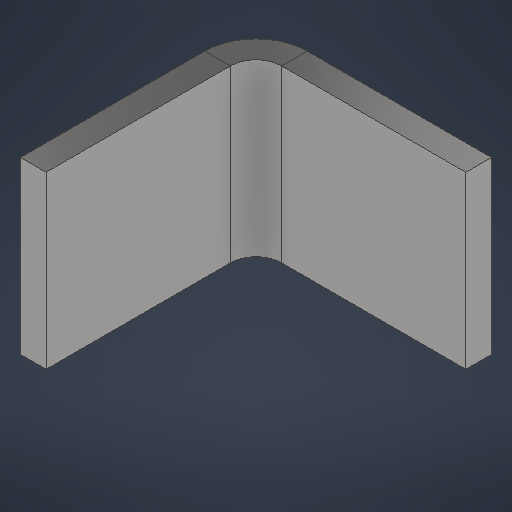
# Autodesk Inventor part: Pressure plate tabs
Saved by Autodesk Inventor 2026.3 (Build 303398000, 398)
## iProperties
Created: 2026-08-04
Part Number: Pressure plate tabs
Material: Generic
Document SubType Name: Sheet Metal
Designer: matot
Density: 1 g/cm^3
Sheet Metal Rule: Default_mm
Appearance: Default
Author: matot
Autodesk Inventor part; units mm, degrees
ref_plane "YZ Plane" through (0, 0, 0) normal (1, 0, 0) x (0, 1, 0)
ref_plane "XZ Plane" through (0, 0, 0) normal (0, 1, 0) x (-1, 0, 0)
ref_plane "XY Plane" through (0, 0, 0) normal (0, 0, 1) x (1, 0, 0)
sketch "Sketch1" plane through (0, 0, 0) normal (1, 0, 0) x (0, 1, 0)
  line L0 (12.963, 18.5185) -> (-7.037, 18.5185)
  line L1 (-7.037, 18.5185) -> (-7.037, -31.4815)
  line L2 (-7.037, -31.4815) -> (12.963, -31.4815)
  line L3 (12.963, -31.4815) -> (12.963, 18.5185)
  point P0 (0, 0)
  dimension "d0" = 50
  dimension "d1" = 20
  measures "d0" distance of L2.end L0.start
  measures "d1" distance of L1.end L2.end
extrude "Plate1" add sketch "Sketch1" along normal blind 3
sketch "Sketch2" plane through (3, 0, 0) normal (1, 0, 0) x (0, 0, -1)
  line L0 (31.4815, 12.963) -> (-18.5185, 12.963) projected
  line L1 (6.4815, 12.963) -> (6.4815, -7.037)
  line L2 (31.4815, -7.037) -> (-18.5185, -7.037) projected
  line L3 (-18.5185, -7.037) -> (-18.5185, 12.963) projected
  point P0 (0, 0)
  dimension "d3" = 20
  dimension "d4" = 25
  constraints: 2 end point, 1 midpoint, 1 perpendicular, 1 vertical
  measures "d3" distance of L1.start L1.end
  measures "d4" distance between parallel lines of L3 L1
fold "Fold1" angle 90 bend radius 3 thickness 3 k factor 0.44 line from (3, 12.963, -6.4815) to (3, -7.037, -6.4815) line at bend centre moving side (0, 0, -1) folds toward (1, 0, 0)
equation "\"d2\" = Thickness"
equation "\"d5\" = BendReliefWidth"
equation "\"d6\" = BendReliefDepth"
equation "\"d7\" = MinimumRemnant"
equation "\"d8\" = TransitionRadius"
equation "\"d10\" = BendRadius"
equation "\"BendRadius\" = Thickness"
equation "\"BendReliefWidth\" = Thickness"
equation "\"BendReliefDepth\" = 0.5 * Thickness"
equation "\"CornerReliefSize\" = 4 * Thickness"
equation "\"MinimumRemnant\" = 2 * Thickness"
equation "\"TransitionRadius\" = BendRadius"
equation "\"JacobiRadiusSize\" = BendRadius"
equation "\"GapSize\" = Thickness"
equation "\"Thickness\" = 3"
body "Solid1"
